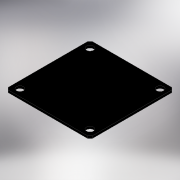
# Autodesk Inventor part: Matek Systems PDU
Saved by Autodesk Inventor 2018 (Build 220112000, 112)
## iProperties
Created: 2018-01-07
Part Number: Matek Systems PDU
Material: GFRC
Document SubType Name: Modeling
Designer: fbl92568
Density: 1.7 g/cm^3
Appearance: Anodized - Black
Author: fbl92568
Autodesk Inventor part; units mm, degrees
ref_plane "YZ Plane" through (0, 0, 0) normal (1, 0, 0) x (0, 1, 0)
ref_plane "XZ Plane" through (0, 0, 0) normal (0, 1, 0) x (-1, 0, 0)
ref_plane "XY Plane" through (0, 0, 0) normal (0, 0, 1) x (1, 0, 0)
sketch "Sketch1" plane through (0, 0, 0) normal (0, 0, 1) x (1, 0, 0)
  line L0 (0, 0) -> (36, 0)
  line L1 (36, 0) -> (36, 36)
  line L2 (36, 36) -> (0, 36)
  line L3 (0, 36) -> (0, 0)
  dimension "d0" = 36
  dimension "d1" = 36
  constraints: 8 end point, 2 parallel, 1 horizontal, 1 perpendicular
  measures "d0" distance of L2.end L1.end
  measures "d1" distance of L1.end L0.end
extrude "Extrusion1" add sketch "Sketch1" along normal blind 1
sketch "Sketch2" plane through (0, 0, 1) normal (0, 0, 1) x (1, 0, 0)
  line L0 (3, 33) -> (33, 33)
  line L1 (33, 33) -> (33, 3)
  line L2 (33, 3) -> (3, 3)
  line L3 (3, 3) -> (3, 33)
  line L4 (0, 36) -> (0, 0) projected
  line L5 (36, 36) -> (0, 36) projected
  circle A0 centre (3, 33) radius 1.525
  circle A1 centre (33, 33) radius 1.525
  circle A2 centre (33, 3) radius 1.525
  circle A3 centre (3, 3) radius 1.525
  dimension "d4" = 30
  dimension "d5" = 30
  dimension "d6" = 3
  dimension "d7" = 3
  dimension "d8" = 3.05
  dimension "d9" = 3.05
  dimension "d10" = 3.05
  dimension "d11" = 3.05
  constraints: 8 end point, 4 centre point, 4 coincident, 2 parallel, 1 horizontal, 1 perpendicular
  measures "d4" distance of L0.start L0.end
  measures "d5" distance of L2.end L0.start
  measures "d6" distance between parallel lines of L4 L3
  measures "d7" distance between parallel lines of L0 L5
  measures "d8" diameter of A0
  measures "d9" diameter of A1
  measures "d10" diameter of A2
  measures "d11" diameter of A3
extrude "Extrusion2" cut sketch "Sketch2" against normal through all contours L3 A0 L0 | L0 A0 L3 | A1 L1 L0 | L0 L1 A1 | A3 L2 L3 | L3 L2 A3 | A2 L2 L1 | L1 L2 A2
chamfer "Chamfer1" distance 1 angle 45 4 edges at (0, 36, 0.5) (36, 36, 0.5) (36, 0, 0.5) (0, 0, 0.5)
body "Solid1"
